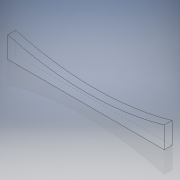
# Autodesk Inventor part: Door retention wall
Saved by Autodesk Inventor 2016 (Build 200138000, 138)
## iProperties
Created: 2017-10-31
Part Number: Door retention wall
Material: Wood (Oak)
Document SubType Name: Modeling
Designer: mathaetaes
Density: 0.76 g/cm^3
Appearance: White Oak - Natural Medium Gloss
Author: mathaetaes
Autodesk Inventor part; units mm, degrees
ref_plane "YZ Plane" through (0, 0, 0) normal (1, 0, 0) x (0, 1, 0)
ref_plane "XZ Plane" through (0, 0, 0) normal (0, 1, 0) x (-1, 0, 0)
ref_plane "XY Plane" through (0, 0, 0) normal (0, 0, 1) x (1, 0, 0)
sketch "Sketch1" plane through (0, 0, 0) normal (0, 0, 1) x (1, 0, 0)
  line L0 (-183.363, 0) -> (186.5245, 0)
  line L1 (186.5245, 0) -> (186.5245, 50.5829)
  line L2 (-183.363, 50.5829) -> (-183.363, 0)
  arc A0 (-183.363, 50.5829) -> (186.5245, 50.5829) centre (1.5807, 702.1816) ccw
  line L3 (-183.363, 50.5829) -> (-183.363, 0)
  line L4 (186.5245, 0) -> (186.5245, 50.5829)
  point P0 (0, 0)
  dimension "d0" = 369.8875
  dimension "d12" = 50.5829
  constraints: 10 end point, 2 point on circle, 1 centre point, 1 horizontal, 1 parallel, 1 perpendicular
  measures "d0" distance of L0.start L0.end
  measures "d12" distance of L0.end L1.end
extrude "Extrusion1" add sketch "Sketch1" along normal blind 19.05
body "Solid1"
